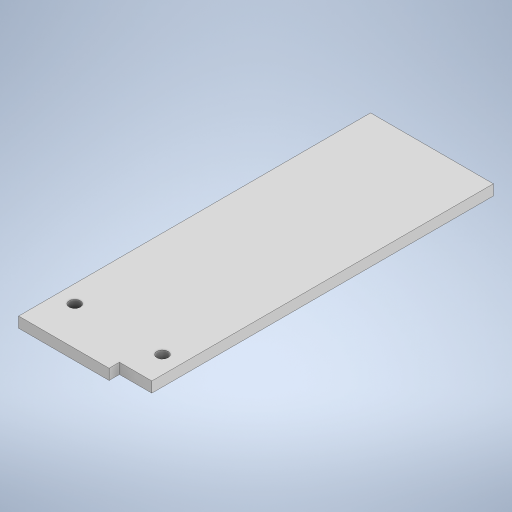
# Autodesk Inventor part: Basis of the robot
Saved by Autodesk Inventor 2023 (Build 270158000, 158)
## iProperties
Created: 2023-05-15
Part Number: Basis of the robot
Material: Типовые
Document SubType Name: Modeling
Designer: ivanc
Density: 1 g/cm^3
Appearance: По умолчанию
Author: ivanc
Autodesk Inventor part; units mm, degrees
ref_plane "YZ Plane" through (0, 0, 0) normal (1, 0, 0) x (0, 1, 0)
ref_plane "XZ Plane" through (0, 0, 0) normal (0, 1, 0) x (-1, 0, 0)
ref_plane "XY Plane" through (0, 0, 0) normal (0, 0, 1) x (1, 0, 0)
sketch "Эскиз1" plane through (0, 0, 0) normal (0, 1, 0) x (-1, 0, 0)
  line L0 (-17.45, 50) -> (17.45, 50)
  line L1 (17.45, 50) -> (17.45, -50)
  line L2 (17.45, -50) -> (-17.45, -50)
  line L3 (-17.45, -50) -> (-17.45, 50)
  line L4 (-17.45, 50) -> (17.45, -50) construction
  line L5 (17.45, 50) -> (-17.45, -50) construction
  line L6 (-17.45, 50) -> (-8.25, 50)
  line L7 (-8.25, 50) -> (-8.25, 47.05)
  line L8 (-8.25, 47.05) -> (-17.45, 47.05)
  line L9 (-17.45, 47.05) -> (-17.45, 50)
  point P0 (0, 0)
  dimension "d0" = 34.9
  dimension "d1" = 100
  dimension "d13" = 9.2
  dimension "d14" = 2.95
  constraints: 20 end point, 4 parallel, 2 horizontal, 2 midpoint, 2 perpendicular
  measures "d0" distance of L1.end L2.end
  measures "d1" distance of L0.end L1.end
  measures "d13" distance of L7.end L8.end
  measures "d14" distance of L6.end L7.end
extrude "Выдавливание1" add sketch "Эскиз1" along normal blind 3 contours L0 L1 L2 L3 L8 L7
sketch "Эскиз2" plane through (0, 3, 0) normal (0, 1, 0) x (1, 0, 0)
  line L0 (-17.45, -50) -> (8.25, -50) projected
  line L1 (0, -50) -> (0, -39.05) construction
  line L2 (-12.45, -39.05) -> (12.45, -39.05)
  point P0 (0, 0)
  point P1 (17.45, -50)
  dimension "d4" = 10.95
  dimension "d5" = 24.9
  constraints: 4 end point, 1 horizontal, 1 midpoint, 1 point on line, 1 vertical
  measures "d4" distance of L1.end L1.start
  measures "d5" distance of L2.start L2.end
hole "Отверстие1" at (12.45, 3, 39.05) at (-12.45, 3, 39.05) direction (0, -1, 0) diameter 3.2 end through all
